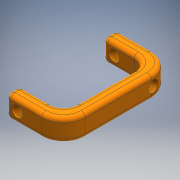
# Autodesk Inventor part: transformer_mount
Saved by Autodesk Inventor 2016 (Build 200138000, 138)
## iProperties
Created: 2016-10-13
Part Number: transformer_mount
Material: Generic
Document SubType Name: Modeling
Designer: Jakub
Density: 1 g/cm^3
Appearance: Default
Mass: 0.553388 g
Surface Area: 6.59593 cm^2
Volume: 0.553388 cm^3
Author: Jakub
Autodesk Inventor part; units mm, degrees
ref_plane "YZ Plane" through (0, 0, 0) normal (1, 0, 0) x (0, 1, 0)
ref_plane "XZ Plane" through (0, 0, 0) normal (0, 1, 0) x (-1, 0, 0)
ref_plane "XY Plane" through (0, 0, 0) normal (0, 0, 1) x (1, 0, 0)
sketch "Sketch1" plane through (0, 0, 0) normal (1, 0, 0) x (0, 1, 0)
  line L0 (-12.5, 2.5) -> (12.5, 2.5)
  line L1 (12.5, 2.5) -> (12.5, -2.5)
  line L2 (12.5, -2.5) -> (-12.5, -2.5)
  line L3 (-12.5, -2.5) -> (-12.5, 2.5)
  line L4 (-12.5, 2.5) -> (12.5, -2.5) construction
  line L5 (12.5, 2.5) -> (-12.5, -2.5) construction
  point P0 (0, 0)
  dimension "d0" = 25
  dimension "d1" = 5
  constraints: 12 end point, 2 midpoint, 2 parallel, 1 horizontal, 1 perpendicular
  measures "d0" distance of L1.end L2.end
  measures "d1" distance of L0.end L1.end
extrude "Extrusion1" add sketch "Sketch1" along normal blind 3
sketch "Sketch2" plane through (0, 0, 0) normal (-1, 0, 0) x (0, 0, 1)
  line L0 (-2.5, -12.5) -> (-2.5, 12.5) projected
  line L1 (2.5, 12.5) -> (2.5, -12.5) projected
  line L2 (-2.5, 12.5) -> (2.5, 12.5)
  line L3 (2.5, 12.5) -> (2.5, 9.5)
  line L4 (2.5, 9.5) -> (-2.5, 9.5)
  line L5 (-2.5, 9.5) -> (-2.5, 12.5)
  line L6 (-2.5, -12.5) -> (2.5, -12.5)
  line L7 (2.5, -12.5) -> (2.5, -9.5)
  line L8 (2.5, -9.5) -> (-2.5, -9.5)
  line L9 (-2.5, -9.5) -> (-2.5, -12.5)
  point P0 (0, 0)
  dimension "d4" = 3
  dimension "d5" = 3
  constraints: 16 end point, 4 parallel, 2 horizontal, 2 perpendicular, 2 point on line
  measures "d4" distance of L2.end L3.end
  measures "d5" distance of L7.end L6.end
extrude "Extrusion2" add sketch "Sketch2" along normal blind 10 contours L0 L8 L1 L6 | L0 L2 L1 L4
fillet "Fillet1" radius 5 2 edges at (3, 12.5, 0) (3, -12.5, 0)
fillet "Fillet2" radius 3 2 edges at (0, 9.5, 0) (0, -9.5, 0)
sketch "Sketch3" plane through (-10, 12.5, 2.5) normal (0, 1, 0) x (1, 0, 0)
  circle A0 centre (2.5, 2.5) radius 1.25
  line L0 (0, 0) -> (0, 5) projected
  line L1 (8, 0) -> (0, 0) projected
  point P0 (10, 2.5)
  dimension "d10" = 2.5
  dimension "d11" = 2.5
  dimension "d12" = 2.5
  constraints: 1 centre point
  measures "d10" diameter of A0
  measures "d11" distance from line of L0 A0.centre
  measures "d12" distance from line of L1 A0.centre
extrude "Extrusion3" cut sketch "Sketch3" against normal through all
fillet "Fillet3" radius 1 4 edges at (-10, 11, 2.5) (-10, 11, -2.5) (-10, -11, 2.5) (-10, -11, -2.5)
fillet "Fillet4" radius 1 32 edges at (-9.7071, 9.5, 2.2071) (-10, 9.5, 0) (-9.7071, 9.5, -2.2071) (-6, 9.5, -2.5) (-0.8787, 8.6213, -2.5) (0, 0, -2.5) (-0.8787, -8.6213, -2.5) (-6, -9.5, -2.5) (-9.7071, -9.5, -2.2071) (-10, -9.5, 0) (-9.7071, -9.5, 2.2071) (-6, -9.5, 2.5) (-0.8787, -8.6213, 2.5) (0, 0, 2.5) (-0.8787, 8.6213, 2.5) (-6, 9.5, 2.5) (-9.7071, 12.5, 2.2071) (-10, 12.5, 0) (-9.7071, 12.5, -2.2071) (-5.5, 12.5, -2.5) (1.5355, 11.0355, -2.5) (3, 0, -2.5) (1.5355, -11.0355, -2.5) (-5.5, -12.5, -2.5) (-9.7071, -12.5, -2.2071) (-10, -12.5, 0) (-9.7071, -12.5, 2.2071) (-5.5, -12.5, 2.5) (1.5355, -11.0355, 2.5) (3, 0, 2.5) (1.5355, 11.0355, 2.5) (-5.5, 12.5, 2.5)
sketch "Sketch4" plane through (3, 0, 0) normal (1, 0, 0) x (0, 0, -1)
  line L0 (0, 0) -> (0, 7.875)
  circle A0 centre (0, 7.875) radius 1.25
  dimension "d17" = 7.875
  dimension "d18" = 2.5
  constraints: 2 end point, 1 centre point, 1 coincident, 1 vertical
  measures "d17" distance of L0.start L0.end
  measures "d18" diameter of A0
extrude "Extrusion4" cut sketch "Sketch4" against normal blind 10
body "Solid1"
